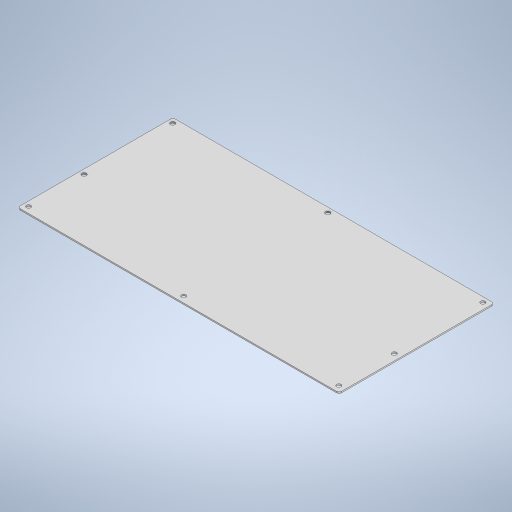
# Autodesk Inventor part: belly pan
Saved by Autodesk Inventor 2023 (Build 270158000, 158)
## iProperties
Created: 2023-11-20
Part Number: belly pan
Material: Generic
Document SubType Name: Modeling
Designer: Robodox
Density: 1 g/cm^3
Appearance: Default
Author: Robodox
Autodesk Inventor part; units mm, degrees
ref_plane "YZ Plane" through (0, 0, 0) normal (1, 0, 0) x (0, 1, 0)
ref_plane "XZ Plane" through (0, 0, 0) normal (0, 1, 0) x (-1, 0, 0)
ref_plane "XY Plane" through (0, 0, 0) normal (0, 0, 1) x (1, 0, 0)
sketch "Sketch1" plane through (0, 0, 0) normal (0, 1, 0) x (-1, 0, 0)
  line L0 (184.15, 101.6) -> (-184.15, 101.6)
  line L1 (-184.15, 101.6) -> (-184.15, -76.2)
  line L2 (-184.15, -76.2) -> (184.15, -76.2)
  line L3 (184.15, -76.2) -> (184.15, 101.6)
  point P0 (0, 0)
  point P1 (0, 0)
  dimension "d0" = 177.8
  dimension "d1" = 368.3
  constraints: 8 end point, 2 parallel, 1 coincident, 1 horizontal, 1 perpendicular
  measures "d0" distance of L2.end L0.start
  measures "d1" distance of L1.end L2.end
extrude "Extrusion1" add sketch "Sketch1" along normal blind 1.5875
sketch "Sketch2" plane through (0, 1.5875, 0) normal (0, 1, 0) x (1, 0, 0)
  circle A0 centre (-178.6621, 70.4533) radius 2.54
  circle A1 centre (176.9379, 70.4533) radius 2.54
  circle A2 centre (-178.6621, -31.1467) radius 2.54
  circle A3 centre (-178.6621, -94.6467) radius 2.54
  circle A4 centre (-0.8621, -94.6467) radius 2.54
  circle A5 centre (176.9379, -31.1467) radius 2.54
  circle A6 centre (176.9379, -94.6467) radius 2.54
  circle A7 centre (-0.8621, 70.4533) radius 2.54
  point P0 (0, 0)
  dimension "d4" = 5.08
  dimension "d6" = 5.08
  dimension "d8" = 5.08
  dimension "d10" = 5.08
  dimension "d12" = 5.08
  dimension "d14" = 5.08
  dimension "d16" = 5.08
  dimension "d17" = 5.08
  constraints: 8 centre point
  measures "d4" diameter of A0
  measures "d6" diameter of A1
  measures "d8" diameter of A2
  measures "d10" diameter of A3
  measures "d12" diameter of A4
  measures "d14" diameter of A5
  measures "d16" diameter of A6
  measures "d17" diameter of A7
extrude "Extrusion2" cut sketch "Sketch2" against normal blind 25.4
fillet "Fillet1" radius 3.175 4 edges at (184.15, 0.7937, 101.6) (184.15, 0.7937, -76.2) (-184.15, 0.7937, -76.2) (-184.15, 0.7937, 101.6)
body "Solid1"
